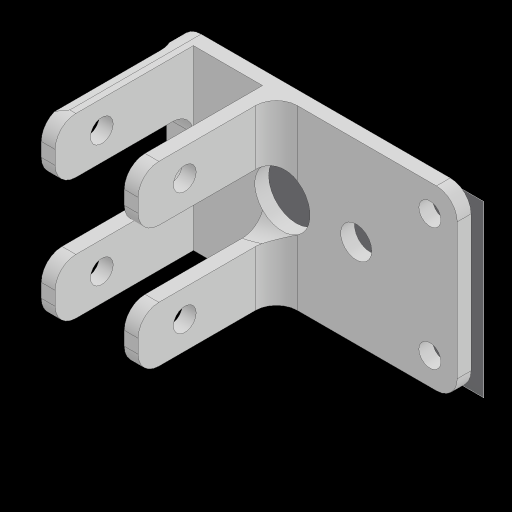
# Autodesk Inventor part: vertMotorHolder
Saved by Autodesk Inventor 2024.3 (Build 283343010, 343A)
## iProperties
Created: 2025-04-13
Part Number: vertMotorHolder
Material: Generic
Document SubType Name: Modeling
Designer: Oleg Kelner
Density: 1 g/cm^3
Appearance: Default
Author: Oleg Kelner
Autodesk Inventor part; units mm, degrees
ref_plane "YZ Plane" through (0, 0, 0) normal (1, 0, 0) x (0, 1, 0)
ref_plane "XZ Plane" through (0, 0, 0) normal (0, 1, 0) x (-1, 0, 0)
ref_plane "XY Plane" through (0, 0, 0) normal (0, 0, 1) x (1, 0, 0)
ref_plane "Work Plane1" through (0, 0, 0) normal (0, 0, 1) x (1, 0, 0)
sketch "Sketch1" plane through (0, 0, 0) normal (0, 0, 1) x (1, 0, 0)
  line L0 (36.7, 22.35) -> (4, 22.35) construction
  arc A0 (4, 22.35) -> (0, 18.35) centre (4, 18.35) ccw construction
  line L1 (0, 4) -> (0, 18.35) construction
  arc A1 (0, 4) -> (4, 0) centre (4, 4) ccw construction
  line L2 (4, 0) -> (36.7, 0) construction
  line L3 (36.7, 0) -> (36.7, 22.35) construction
  circle A2 centre (32.75, 2.3) radius 1.5 construction
  circle A3 centre (32.75, 20.05) radius 1.5 construction
  circle A4 centre (22.095, 11.175) radius 1.915 construction
  circle A5 centre (11.43, 11.175) radius 3.5 construction
  line L4 (0, 8.725) -> (0, 13.625) construction
  line L5 (0, 13.625) -> (-4.65, 13.625) construction
  line L6 (-4.65, 13.625) -> (-4.65, 8.725) construction
  line L7 (-4.65, 8.725) -> (0, 8.725) construction
  circle A6 centre (-2.325, 11.175) radius 1.445 construction
  circle A7 centre (32.75, 20.05) radius 1.6
  circle A8 centre (32.75, 2.3) radius 1.6
  circle A9 centre (-2.325, 11.175) radius 1.15
  circle A10 centre (32.75, 20.05) radius 3.95 construction
  circle A11 centre (32.75, 2.3) radius 3.95 construction
  line L8 (36.7, 24) -> (36.7, -1.65)
  line L9 (36.7, -1.65) -> (-5.325, -1.65)
  line L10 (-5.325, -1.65) -> (-5.325, 24)
  line L11 (-5.325, 24) -> (36.7, 24)
  circle A12 centre (22.095, 11.175) radius 2.25
  circle A13 centre (11.43, 11.175) radius 4
  point P0 (0, 0)
  point P1 (36.7, 11.175)
  point P2 (-5.325, 11.175)
  dimension "d0" = 3.2
  dimension "d1" = 3.2
  dimension "d2" = 2.3
  dimension "d3" = 3
  dimension "d4" = 4.5
  dimension "d5" = 8
  constraints: 8 end point, 7 centre point, 7 coincident, 3 midpoint, 3 tangent, 2 parallel, 2 perpendicular
  measures "d0" diameter of A7
  measures "d1" diameter of A8
  measures "d2" diameter of A9
  measures "d3" distance of A6.centre point (-5.325, 11.175)
  measures "d4" diameter of A12
  measures "d5" diameter of A13
extrude "Extrusion1" add sketch "Sketch1" along normal blind 2
sketch "Sketch2" plane through (0, 0, 2) normal (0, 0, 1) x (1, 0, 0)
  line L0 (8.555, 43.93) -> (8.555, -55.1648) construction
  line L1 (8.555, -55.1648) -> (-1.445, -55.1648) construction
  line L2 (-1.445, 43.93) -> (-1.445, -55.1648) construction
  line L3 (8.555, 43.93) -> (-1.445, 43.93) construction
  line L4 (36.7, 24) -> (-5.325, 24) construction
  line L5 (8.555, 24) -> (8.555, 16)
  line L6 (8.555, 16) -> (10.555, 16)
  line L7 (10.555, 16) -> (10.555, 24)
  line L8 (10.555, 24) -> (8.555, 24)
  line L9 (-5.325, -1.65) -> (36.7, -1.65) construction
  line L10 (8.555, -1.65) -> (8.555, 6.35)
  line L11 (8.555, 6.35) -> (10.555, 6.35)
  line L12 (10.555, 6.35) -> (10.555, -1.65)
  line L13 (10.555, -1.65) -> (8.555, -1.65)
  line L14 (-1.445, 24) -> (-1.445, 16)
  line L15 (-1.445, 16) -> (-3.445, 16)
  line L16 (-3.445, 16) -> (-3.445, 24)
  line L17 (-3.445, 24) -> (-1.445, 24)
  line L18 (-1.445, -1.65) -> (-1.445, 6.35)
  line L19 (-1.445, 6.35) -> (-3.445, 6.35)
  line L20 (-3.445, 6.35) -> (-3.445, -1.65)
  line L21 (-3.445, -1.65) -> (-1.445, -1.65)
  point P0 (0, 0)
  dimension "d8" = 8
  dimension "d9" = 2
  dimension "d10" = 8
  dimension "d11" = 2
  dimension "d12" = 2
  dimension "d13" = 8
  dimension "d14" = 2
  dimension "d15" = 8
  constraints: 32 end point, 12 point on line, 8 parallel, 4 perpendicular
  measures "d8" distance of L5.start L5.end
  measures "d9" distance of L6.end L5.end
  measures "d10" distance of L10.start L10.end
  measures "d11" distance of L10.end L11.end
  measures "d12" distance of L14.end L15.end
  measures "d13" distance of L18.start L18.end
  measures "d14" distance of L19.end L18.end
  measures "d15" distance between parallel lines of L17 L15
extrude "Extrusion2" add sketch "Sketch2" along normal blind 20
fillet "Fillet1" radius 3 6 edges at (-2.445, 16, 2) (-2.445, 6.35, 2) (-3.445, 2.35, 2) (-3.445, 20, 2) (10.555, 20, 2) (10.555, 2.35, 2)
fillet "Fillet3" radius 3 2 edges at (11.055, 16, 2) (11.055, 6.35, 2)
fillet "Fillet4" radius 3 12 edges at (9.555, 24, 22) (9.555, 16, 22) (-2.445, 24, 22) (-2.445, 16, 22) (9.555, 6.35, 22) (9.555, -1.65, 22) (-2.445, 6.35, 22) (-2.445, -1.65, 22) (36.7, -1.65, 1) (36.7, 24, 1) (-5.325, 24, 1) (-5.325, -1.65, 1)
sketch "Sketch3" plane through (10.555, -1.65, 5) normal (1, 0, 0) x (0, 0, -1)
  line L0 (-17, 20.65) -> (-17, 22.65) projected
  line L1 (-3.5, 45.58) -> (-3.5, -53.5148) projected
  line L2 (0, 25.65) -> (-14, 25.65) projected
  line L3 (0, 8) -> (-14, 8) projected
  line L4 (-17, 3) -> (-17, 5) projected
  point P0 (5, 1.65)
  point P1 (-10.25, 21.65)
  point P2 (-17, 21.65)
  point P3 (-17, 21.65)
  point P4 (-10.25, 4)
  point P5 (-17, 4)
  dimension "d22" = 6.75
  dimension "d24" = 4
  dimension "d25" = 4
  dimension "d26" = 6.75
  constraints: 3 midpoint
  measures "d22" distance of point (-17, 21.65) point (-10.25, 21.65)
  measures "d24" distance from line of L2 point (-10.25, 21.65)
  measures "d25" distance from line of L3 point (-10.25, 4)
  measures "d26" distance of point (-10.25, 4) point (-17, 4)
hole "Hole1" at (10.555, 20, 15.25) at (10.555, 2.35, 15.25) direction (-1, 0, 0) diameter 3.3 depth 14
body "Solid1"
